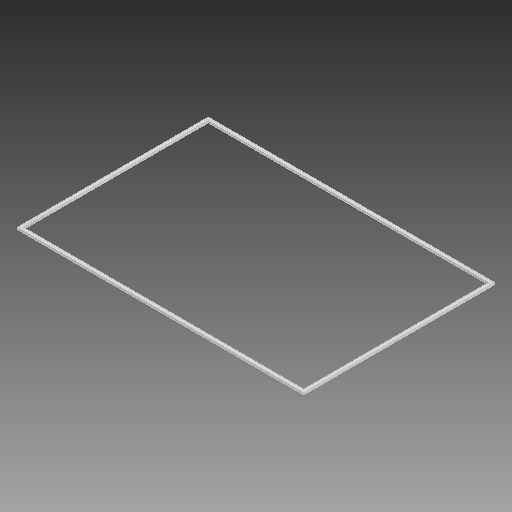
# Autodesk Inventor part: Playing_place
Saved by Autodesk Inventor 2023 (Build 270158000, 158)
## iProperties
Created: 2022-01-17
Part Number: Playing_place
Material: Типовые
Document SubType Name: Modeling
Designer: Администратор
Density: 1 g/cm^3
Appearance: По умолчанию
Author: Администратор
Autodesk Inventor part; units mm, degrees
ref_plane "YZ Plane" through (0, 0, 0) normal (1, 0, 0) x (0, 1, 0)
ref_plane "XZ Plane" through (0, 0, 0) normal (0, 1, 0) x (-1, 0, 0)
ref_plane "XY Plane" through (0, 0, 0) normal (0, 0, 1) x (1, 0, 0)
sketch "Эскиз1" plane through (0, 0, 0) normal (0, 1, 0) x (-1, 0, 0)
  line L0 (915, -610) -> (-915, -610)
  line L1 (-915, -610) -> (-915, 610)
  line L2 (-915, 610) -> (915, 610)
  line L3 (915, 610) -> (915, -610)
  line L4 (0, -610) -> (0, 610) construction
  line L5 (915, 0) -> (-915, 0) construction
  line L6 (-895, -590) -> (895, -590)
  line L7 (895, -590) -> (895, 590)
  line L8 (895, 590) -> (-895, 590)
  line L9 (-895, 590) -> (-895, -590)
  line L10 (895, -300) -> (915, -300)
  line L11 (895, 300) -> (915, 300)
  line L12 (-895, -300) -> (-915, -300)
  line L13 (-895, 300) -> (-915, 300)
  line L14 (-895, -450) -> (-595, -450)
  line L15 (-595, -450) -> (-595, 450)
  line L16 (-595, 450) -> (-895, 450)
  line L17 (-895, 430) -> (-615, 430)
  line L18 (-615, 430) -> (-615, -430)
  line L19 (-615, -430) -> (-895, -430)
  line L20 (895, -450) -> (595, -450)
  line L21 (595, -450) -> (595, 450)
  line L22 (595, 450) -> (895, 450)
  line L23 (895, 430) -> (615, 430)
  line L24 (615, 430) -> (615, -430)
  line L25 (615, -430) -> (895, -430)
  point P0 (0, 0)
  point P1 (0, 0)
  dimension "d0" = 1830
  dimension "d1" = 1220
  dimension "d2" = 20
  dimension "d8" = 600
  dimension "d9" = 900
  dimension "d10" = 300
  dimension "d11" = 20
  constraints: 52 end point, 12 symmetric about line, 7 perpendicular, 6 point on line, 5 midpoint, 4 parallel, 2 horizontal, 1 coincident, 7 other
  measures "d0" distance of L0.start L0.end
  measures "d1" distance of L2.end L0.start
  measures "d2" distance between parallel lines of L0 L6
  measures "d8" distance between parallel lines of L10 L11
  measures "d9" distance of L14.end L15.end
  measures "d10" distance of L14.start L14.end
  measures "d11" distance between parallel lines of L15 L18
extrude "Выдавливание1" add sketch "Эскиз1" along normal blind 12 contours L0 L1 L12 L9 L6 L7 L10 L3 | L10 L7 L11 L3 | L1 L13 L9 L12 | L11 L7 L8 L9 L13 L1 L2 L3
